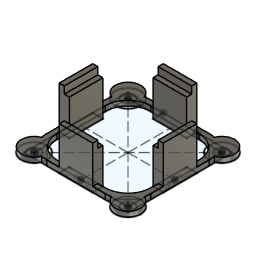
Bracket_holder_v2 (Autodesk Fusion 360 design; units mm, degrees)
Autodesk Fusion 360 part; units mm, degrees
sketch "Sketch1" plane through (0, 0, 0) normal (0, 0, 1) x (1, 0, 0)
  line L0 (0, 0) -> (92.5, 0)
  line L1 (92.5, 0) -> (92.5, 92.5)
  line L2 (92.5, 92.5) -> (0, 92.5)
  line L3 (0, 92.5) -> (0, 0)
  line L4 (-5, -5) -> (97.5, -5)
  line L5 (97.5, -5) -> (97.5, 97.5)
  line L6 (97.5, 97.5) -> (-5, 97.5)
  line L7 (-5, 97.5) -> (-5, -5)
  line L8 (0, 0) -> (92.5, 92.5) construction
  line L9 (92.5, 0) -> (0, 92.5) construction
  line L10 (46.25, 46.25) -> (92.5, 46.25) construction
  line L11 (46.25, 46.25) -> (46.25, 92.5) construction
  line L12 (46.25, 46.25) -> (0, 46.25) construction
  line L13 (46.25, 46.25) -> (46.25, 0) construction
  line L14 (97.5, 29.75) -> (87.5, 29.75)
  line L15 (87.5, 29.75) -> (87.5, 62.75)
  line L16 (87.5, 62.75) -> (97.5, 62.75)
  line L17 (97.5, 62.75) -> (97.5, 29.75)
  line L18 (97.5, 29.75) -> (87.5, 62.75) construction
  line L19 (87.5, 29.75) -> (97.5, 62.75) construction
  line L20 (62.75, -5) -> (29.75, -5)
  line L21 (29.75, -5) -> (29.75, 5)
  line L22 (29.75, 5) -> (62.75, 5)
  line L23 (62.75, 5) -> (62.75, -5)
  line L24 (62.75, -5) -> (29.75, 5) construction
  line L25 (29.75, -5) -> (62.75, 5) construction
  line L26 (5, 29.75) -> (5, 62.75)
  line L27 (5, 62.75) -> (-5, 62.75)
  line L28 (-5, 62.75) -> (-5, 29.75)
  line L29 (-5, 29.75) -> (5, 29.75)
  line L30 (62.75, 87.5) -> (62.75, 97.5)
  line L31 (29.75, 87.5) -> (62.75, 87.5)
  line L32 (29.75, 97.5) -> (29.75, 87.5)
  circle A0 centre (0, 92.5) radius 12.5
  circle A1 centre (92.5, 92.5) radius 12.5
  circle A2 centre (0, 0) radius 12.5
  circle A3 centre (92.5, 0) radius 12.5
  line L33 (0, 12.5) -> (12.5, 0)
  line L34 (80, 0) -> (92.5, 12.5)
  line L35 (80, 92.5) -> (92.5, 80)
  line L36 (12.5, 92.5) -> (0, 80)
  circle A4 centre (0, 0) radius 6
  circle A5 centre (92.5, 0) radius 6
  circle A6 centre (92.5, 92.5) radius 6
  circle A7 centre (0, 92.5) radius 6
  point P0 (92.5, 46.25)
  point P1 (46.25, 0)
  dimension "d1" = 92.5
  dimension "d2" = 92.5
  dimension "d3" = 5
  dimension "d4" = 10
  dimension "d5" = 33
  dimension "d6" = 33
  dimension "d7" = 10
  dimension "d18" = 25
  dimension "d19" = 25
  dimension "d20" = 25
  dimension "d21" = 25
  dimension "d24" = 12
  dimension "d25" = 12
  dimension "d26" = 12
  dimension "d27" = 12
  constraint horizontal L0
  constraint vertical L1
  constraint horizontal L2
  constraint vertical L3
  constraint coincident L0.start L3.end
  constraint midpoint L9 L10.start
  constraint midpoint L1 P0
  constraint midpoint L2 L11.end
  constraint midpoint L3 L12.end
  constraint midpoint L0 P1
  constraint horizontal L14
  constraint perpendicular L14 L15
  constraint parallel L14 L16
  constraint parallel L15 L17
  constraint coincident L18 P0
  constraint coincident L19 P0
  constraint coincident P0 L10.end
  constraint horizontal L20
  constraint perpendicular L20 L21
  constraint parallel L20 L22
  constraint parallel L21 L23
  constraint coincident L24 P1
  constraint coincident L25 P1
  constraint coincident P1 L13.end
  constraint symmetric L11 L14.start L28.end
  constraint symmetric L11 L14.end L26.start
  constraint symmetric L11 L15.end L26.end
  constraint symmetric L11 L16.end L27.end
  constraint symmetric L10 L20.start L30.end
  constraint symmetric L10 L20.end L32.start
  constraint symmetric L10 L21.end L31.start
  constraint symmetric L10 L22.end L30.start
  constraint coincident L2.end L3.start
  constraint coincident L1.end L2.start
  constraint coincident L0.end L1.start
  constraint coincident L3 L33.start
  constraint coincident A2 L33.start
  constraint coincident L0 L33.end
  constraint coincident A2 L33.end
  constraint coincident A3 L34.start
  constraint coincident L0 L34.start
  constraint coincident A3 L34.end
  constraint coincident L1 L34.end
  constraint coincident A1 L35.start
  constraint coincident L2 L35.start
  constraint coincident A1 L35.end
  constraint coincident L1 L35.end
  constraint coincident A0 L36.start
  constraint coincident L2 L36.start
  constraint coincident A0 L36.end
  constraint coincident L3 L36.end
  constraint concentric A2 A4
  constraint concentric A3 A5
  constraint concentric A1 A6
  constraint concentric A0 A7
  measures "d1" distance of L0.start L0.end
  measures "d2" distance of L0 L2
  measures "d4" distance of L15.end L16.end
  measures "d5" distance of L14.end L15.end
  measures "d6" distance of L21.end L22.end
  measures "d7" distance of L20.end L21.end
  measures "d18" diameter of A1
  measures "d19" diameter of A0
  measures "d20" diameter of A2
  measures "d21" diameter of A3
  measures "d24" diameter of A4
  measures "d25" diameter of A5
  measures "d26" diameter of A6
  measures "d27" diameter of A7
extrude "Extrude1" add sketch "Sketch1" along normal blind 5 contours L0 L3 L4 L7 A4 | L0 L4 A2 A4 | L3 L7 A2 A4 | L0 L4 L21 A2 | L3 L7 L29 A2 | L0 L21 L22 L23 | L0 L4 L20 L21 L23 | L4 L7 A4 | L3 L7 L27 L28 L29 | L3 L26 L27 L29 | L0 L4 L23 A3 | L3 L7 L27 A0 | L0 L4 A3 A5 | L3 L7 A0 A7 | L0 L1 L4 L5 A5 | L1 L5 A3 A5 | L1 L5 L14 A3 | L2 L3 L6 L7 A7 | L2 L6 L32 A0 | L2 L6 A0 A7 | L1 L14 L15 L16 | L1 L5 L14 L16 L17 | L2 L6 L30 L32 | L2 L30 L31 L32 | L4 L5 A5 | L1 L5 L16 A1 | L6 L7 A7 | L2 L6 L30 A1 | L1 L5 A1 A6 | L2 L6 A1 A6 | L1 L2 L5 L6 A6 | L5 L6 A6
extrude "Extrude2" add sketch "Sketch1" along normal blind 30 from surface at 5 contours L0 L21 L22 L23 | L0 L4 L20 L21 L23 | L3 L7 L27 L28 L29 | L3 L26 L27 L29 | L1 L14 L15 L16 | L1 L5 L14 L16 L17 | L2 L6 L30 L32 | L2 L30 L31 L32
extrude "Extrude3" add sketch "Sketch1" along normal blind 7 from surface at 35 contours L0 L4 L20 L21 L23 | L3 L7 L27 L28 L29 | L1 L5 L14 L16 L17 | L2 L6 L30 L32
fillet "Fillet1" radius 22.5 8 edges at (92.5, 92.5, 2.5) (97.5, 97.5, 2.5) (0, 92.5, 2.5) (-5, 97.5, 2.5) (-5, -5, 2.5) (0, 0, 2.5) (92.5, 0, 2.5) (97.5, -5, 2.5)
extrude "Extrude4" add sketch "Sketch1" along normal blind 5 contours L0 L3 A4 | L0 L3 L4 L7 A4 | L0 L3 L33 A4 | L0 L4 A2 A4 | L3 L7 A2 A4 | L4 A4 | L4 L7 A2 A4 | L7 A4 | L4 L7 A4 | L0 L1 L34 A5 | L0 L4 A3 A5 | L3 L7 A0 A7 | L2 L3 L36 A7 | L0 L1 A5 | L0 L1 L4 L5 A5 | L1 L5 A3 A5 | L4 L5 A3 A5 | L2 L3 L6 L7 A7 | L2 L3 A7 | L2 L6 A0 A7 | L6 L7 A0 A7 | L4 A5 | L7 A7 | L5 A5 | L4 L5 A5 | L6 L7 A7 | L6 A7 | L1 L2 L35 A6 | L1 L5 A1 A6 | L2 L6 A1 A6 | L1 L2 A6 | L1 L2 L5 L6 A6 | L5 L6 A1 A6 | L5 A6 | L6 A6 | L5 L6 A6
extrude "Extrude5" cut sketch "Sketch1" along normal blind 2 contours L0 L3 A4 | L0 L3 L4 L7 A4 | L4 A4 | L7 A4 | L0 L1 A5 | L0 L1 L4 L5 A5 | L2 L3 L6 L7 A7 | L2 L3 A7 | L4 A5 | L7 A7 | L5 A5 | L6 A7 | L1 L2 A6 | L1 L2 L5 L6 A6 | L5 A6 | L6 A6
